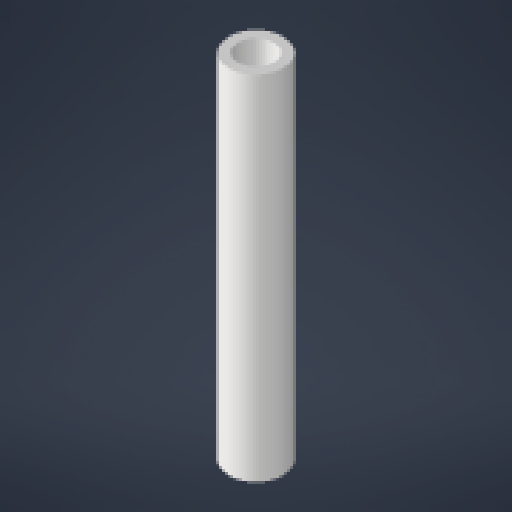
# Autodesk Inventor part: GasEinlass_Flansch
Saved by Autodesk Inventor 2027 (Build 310192060, 192F)
## iProperties
Created: 2026-08-01
Part Number: GasEinlass_Flansch
Material: Generic
Document SubType Name: Modeling
Designer: kw
Density: 1 g/cm^3
Appearance: Default
Author: kw
Autodesk Inventor part; units mm, degrees
ref_plane "YZ Plane" through (0, 0, 0) normal (1, 0, 0) x (0, 1, 0)
ref_plane "XZ Plane" through (0, 0, 0) normal (0, 1, 0) x (-1, 0, 0)
ref_plane "XY Plane" through (0, 0, 0) normal (0, 0, 1) x (1, 0, 0)
sketch "Sketch1" plane through (0, 0, 0) normal (0, 1, 0) x (-1, 0, 0)
  circle A0 centre (0, 0) radius 1
  circle A1 centre (0, 0) radius 1.55
  dimension "d0" = 2
  dimension "d1" = 3.1
  constraints: 2 centre point, 2 coincident
  measures "d0" diameter of A0
  measures "d1" diameter of A1
extrude "Extrusion1" add sketch "Sketch1" along normal blind 20
body "Solid1"
